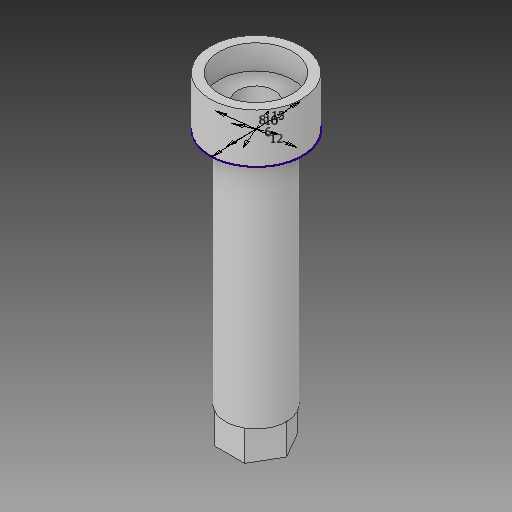
# Autodesk Inventor part: vacuum-gear-shaft
Saved by Autodesk Inventor 2017 (Build 210142000, 142)
## iProperties
Created: 2026-03-25
Part Number: vacuum-gear-shaft
Material: Generic
Document SubType Name: Modeling
Designer: a
Density: 1 g/cm^3
Appearance: Default
Author: a
Autodesk Inventor part; units mm, degrees
ref_plane "YZ Plane" through (0, 0, 0) normal (1, 0, 0) x (0, 1, 0)
ref_plane "XZ Plane" through (0, 0, 0) normal (0, 1, 0) x (-1, 0, 0)
ref_plane "XY Plane" through (0, 0, 0) normal (0, 0, 1) x (1, 0, 0)
sketch "Sketch1" plane through (0, 0, 0) normal (0, 1, 0) x (-1, 0, 0)
  circle A0 centre (0, 0) radius 7.5
  circle A1 centre (0, 0) radius 5
  circle A2 centre (0, 0) radius 4
  circle A3 centre (0, 0) radius 3
  circle A4 centre (0, 0) radius 6
  dimension "d0" = 15
  dimension "d1" = 10
  dimension "d2" = 8
  dimension "d7" = 6
  dimension "d8" = 12
  constraints: 5 centre point, 5 coincident
  measures "d0" diameter of A0
  measures "d1" diameter of A1
  measures "d2" diameter of A2
  measures "d7" diameter of A3
  measures "d8" diameter of A4
extrude "Extrusion1" add sketch "Sketch1" along normal blind 8 contours A0
extrude "Extrusion2" add sketch "Sketch1" against normal blind 44 contours A1 | A2
extrude "Extrusion3" add sketch "Sketch1" along normal blind 4 contours A0 | A1 | A2 | A4
sketch "Sketch2" plane through (0, -44, 0) normal (0, -1, 0) x (1, 0, 0)
  circle A0 centre (0, 0) radius 5 projected
  line L0 (5, 0) -> (2.5, -4.3301)
  line L1 (2.5, -4.3301) -> (-2.5, -4.3301)
  line L2 (-2.5, -4.3301) -> (-5, 0)
  line L3 (-5, 0) -> (-2.5, 4.3301)
  line L4 (-2.5, 4.3301) -> (2.5, 4.3301)
  line L5 (2.5, 4.3301) -> (5, 0)
  circle A1 centre (0, 0) radius 5
  dimension "d11" = 10
  constraints: 12 end point, 2 coincident, 1 centre point, 1 horizontal alignment, 14 other
  measures "d11" diameter of A1
extrude "Extrusion4" cut sketch "Sketch2" against normal blind 5 contours L5 A0 | A0 L0 | L4 A0 | A0 L1 | L3 A0 | A0 L2
body "Solid1"
